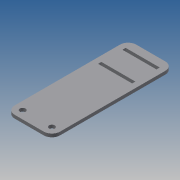
# Autodesk Inventor part: ribbon slider manager
Saved by Autodesk Inventor 2013 (Build 170138000, 138)
## iProperties
Created: 2017-04-10
Part Number: ribbon slider manager
Material: Generic
Document SubType Name: Modeling
Designer: employee
Density: 1 g/cm^3
Author: employee
Autodesk Inventor part; units mm, degrees
ref_plane "YZ Plane" through (0, 0, 0) normal (1, 0, 0) x (0, 1, 0)
ref_plane "XZ Plane" through (0, 0, 0) normal (0, 1, 0) x (-1, 0, 0)
ref_plane "XY Plane" through (0, 0, 0) normal (0, 0, 1) x (1, 0, 0)
sketch "Sketch1" plane through (0, 0, 0) normal (0, 0, 1) x (1, 0, 0)
  line L0 (-14, 0) -> (14, 0)
  line L1 (14, 0) -> (14, 75)
  line L2 (14, 75) -> (-14, 75)
  line L3 (-14, 75) -> (-14, 0)
  circle A0 centre (-9, 5) radius 1.75
  circle A1 centre (9, 5) radius 1.75
  line L4 (-9, 5) -> (9, 5)
  point P0 (0, 0)
  point P1 (0, 0)
  point P2 (0, 5)
  dimension "d0" = 75
  dimension "d2" = 28
  dimension "d3" = 5
  dimension "d4" = 3.5
  dimension "d5" = 18
  constraints: 10 end point, 2 centre point, 2 horizontal, 2 midpoint, 2 parallel, 1 coincident, 1 equal radius, 1 perpendicular, 1 vertical alignment
  measures "d0" distance of L0.end L1.end
  measures "d2" distance of L0.start L0.end
  measures "d3" distance between parallel lines of L4 L0
  measures "d4" diameter of A1
  measures "d5" distance of L4.start L4.end
extrude "Extrusion1" add sketch "Sketch1" along normal blind 2
sketch "Sketch4" plane through (0, 0, 2) normal (0, 0, 1) x (1, 0, 0)
  line L0 (14, 75) -> (-14, 75) projected
  line L1 (-10.5, 70) -> (10.5, 70)
  line L2 (10.5, 70) -> (10.5, 68)
  line L3 (10.5, 68) -> (-10.5, 68)
  line L4 (-10.5, 68) -> (-10.5, 70)
  line L5 (-10.5, 53) -> (10.5, 53)
  line L6 (10.5, 53) -> (10.5, 55)
  line L7 (10.5, 55) -> (-10.5, 55)
  line L8 (-10.5, 55) -> (-10.5, 53)
  point P0 (0, 0)
  point P1 (0, 53)
  point P2 (0, 68)
  point P3 (0, 75)
  dimension "d19" = 21
  dimension "d21" = 2
  dimension "d22" = 5
  dimension "d23" = 15
  constraints: 16 end point, 4 parallel, 3 midpoint, 2 equal length, 2 horizontal, 2 perpendicular, 2 vertical alignment
  measures "d19" distance of L1.start L1.end
  measures "d21" distance of L1.end L2.end
  measures "d22" distance between parallel lines of L0 L1
  measures "d23" distance between parallel lines of L7 L1
extrude "Extrusion4" cut sketch "Sketch4" against normal through all
fillet "Fillet2" radius 5 4 edges at (14, 75, 1) (-14, 75, 1) (14, 0, 1) (-14, 0, 1)
sketch "Sketch2" plane through (0, 0, 2) normal (0, 0, 1) x (1, 0, 0)
  line L0 (14, 75) -> (-14, 75) projected
  line L1 (-11, 75) -> (11, 75)
  line L2 (11, 75) -> (11, 65)
  line L3 (11, 65) -> (-11, 65)
  line L4 (-11, 65) -> (-11, 75)
  line L5 (-11, 65) -> (-14, 65)
  line L6 (-14, 65) -> (-14, 75)
  line L7 (-14, 75) -> (-11, 75)
  line L8 (-11, 75) -> (-11, 65)
  line L9 (11, 65) -> (14, 65)
  line L10 (14, 65) -> (14, 75)
  line L11 (14, 75) -> (11, 75)
  line L12 (11, 75) -> (11, 65)
  point P0 (0, 0)
  point P1 (0, 75)
  dimension "d8" = 10
  dimension "d10" = 22
  constraints: 24 end point, 6 parallel, 3 horizontal, 3 perpendicular, 2 midpoint, 1 point on line
  measures "d8" distance of L1.end L2.end
  measures "d10" distance between parallel lines of L2 L4
sketch "Sketch3" plane through (0, 0, 4) normal (0, 0, 1) x (1, 0, 0)
  line L0 (-11, 65) -> (-11, 75) projected
  line L1 (-11, 75) -> (-14, 75) projected
  line L2 (-14, 75) -> (-14, 65) projected
  line L3 (-14, 65) -> (-11, 65) projected
  line L4 (14, 75) -> (11, 75) projected
  line L5 (11, 75) -> (11, 65) projected
  line L6 (11, 65) -> (14, 65) projected
  line L7 (14, 65) -> (14, 75) projected
  line L8 (-11, 75) -> (11, 75)
  line L9 (11, 75) -> (11, 65)
  line L10 (11, 65) -> (-11, 65)
  line L11 (-11, 65) -> (-11, 75)
  point P0 (0, 0)
  constraints: 8 end point, 2 parallel, 1 horizontal, 1 perpendicular
body "Solid1"
